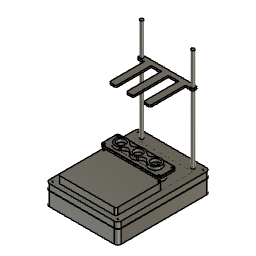
group 5 (Autodesk Fusion 360 design; units mm, degrees)
Autodesk Fusion 360 part; units mm, degrees
note: some values were not read from the file. Chosen so that the rebuilt part matches the saved one: which face or edge a step refers to.
(part 1 of 2)
sketch "Sketch1" plane through (0, 0, 0) normal (0, 0, 1) x (1, 0, 0)
  line L0 (127.613, 86.765) -> (0.7281, 86.765)
  line L1 (127.613, 0.765) -> (127.613, 86.765)
  line L2 (0.7281, 0.765) -> (127.613, 0.765)
  line L3 (0.7281, 86.765) -> (0.7281, 0.765)
  dimension "d1" = 86
  dimension "d2" = 126.8849
  constraint horizontal L0
  constraint vertical L3
  constraint horizontal L2
  constraint vertical L1
  measures "d1" distance of L2.start L0.end
  measures "d2" distance of L0.start L0.end
extrude "Extrude1" add sketch "Sketch1" along normal blind 30 makes body 1
sketch "Sketch2" plane through (0, 0, 30) normal (0, 0, 1) x (-1, 0, 0)
  line L0 (-0.7281, -86.765) -> (-0.7281, -0.765)
  line L1 (-0.7281, -0.765) -> (-127.613, -0.765)
  line L2 (-127.613, -0.765) -> (-127.613, -86.765)
  line L3 (-127.613, -86.765) -> (-0.7281, -86.765)
  circle A0 centre (-30, -70) radius 10
  circle A1 centre (-60, -70) radius 10
  circle A2 centre (-90, -70) radius 10
  circle A3 centre (-30, -30) radius 10
  circle A4 centre (-60, -30) radius 10
  circle A5 centre (-90, -30) radius 10
  point P0 (-30, -70)
  dimension "d5" = 20
  dimension "d6" = 20
  dimension "d7" = 20
  dimension "d8" = 20
  measures "d5" diameter of A2
  measures "d6" diameter of A3
  measures "d7" diameter of A4
  measures "d8" diameter of A5
extrude "Extrude2" cut sketch "Sketch2" against normal blind 10 contours A0 | A1 | A2 | A3 | A4 | A5 bodies 1
sketch "Sketch3" plane through (0, 0, 0) normal (0, 0, 1) x (1, 0, 0)
  circle A0 centre (23.2455, 19.8373) radius 15
  dimension "d11" = 30
  measures "d11" diameter of A0
extrude "Extrude3" add sketch "Sketch3" against normal blind 10 bodies 1
move_face "MoveFace1" to x (1, 0, 0) y (0, 1, 0) z (0, 0, 1) at (0, 0, -20) 1 faces at (38.2269, 19.0896, -6.6667) on bodies 1
move_face "MoveFace2" to x (1, 0, 0) y (0, 1, 0) z (0, 0, 1) at (0, 0, -10) 1 faces at (38.2269, 19.0896, -6.6667) on bodies 1
move_face "MoveFace3" by (0, 0, -15) 1 faces at (27.3111, 19.0921, -10) on bodies 1
move_face "MoveFace4" to x (1, 0, 0) y (0, 1, 0) z (0, 0, 1) at (0, 0, -15) 1 faces at (38.2269, 19.0896, -16.6667) on bodies 1
move_face "MoveFace5" to x (1, 0, 0) y (0, 1, 0) z (0, 0, 1) at (0, 0, -10) 1 faces at (38.2269, 19.0896, -16.6667) on bodies 1
move_face "MoveFace6" to x (1, 0, 0) y (0, 1, 0) z (0, 0, 1) at (0, 0, 15) 1 faces at (38.2269, 19.0896, -16.6667) on bodies 1
split "Split1" by plane through (0, 0, 0) normal (0, 0, -1) bodies 1 makes body 2 at (38.171, 18.3438, -8.3333)
move_face "MoveFace7" to x (1, 0, 0) y (0, 1, 0) z (0, 0, 1) at (0, 0, -20) 1 faces at (38.171, 18.3438, -8.3333) on bodies 2
move_face "MoveFace8" to x (1, 0, 0) y (0, 1, 0) z (0, 0, 1) at (120, 0, -10) 1 faces at (38.171, 18.3438, -8.3333) on bodies 2
extrude "Extrude4" cut 1 faces at (147.3111, 20.5825, 0) along direction (0, 0, -1) blind 10 on bodies 2 bodies 2
move_face "MoveFace9" to x (1, 0, 0) y (0, 1, 0) z (0, 0, 1) at (0, 0, -10) 1 faces at (158.171, 18.3438, -20) on bodies 2
move_body "Move1" bodies 2 to x (1, 0, 0) y (0, 1, 0) z (0, 0, 1) at (0, 0, -20)
sketch "Sketch4" plane through (0, 0, -30) normal (0, 0, 1) x (-1, 0, 0)
  circle A0 centre (-143.2455, -19.8373) radius 15
  circle A1 centre (-143.2455, -19.8373) radius 1
  dimension "d16" = 2
  constraint concentric A0 A1
  measures "d16" diameter of A1
extrude "Extrude5" add sketch "Sketch4" along normal blind 7 contours A1 bodies 2
sketch "Sketch5" plane through (0, 0, -23) normal (0, 0, 1) x (-1, 0, 0)
  circle A0 centre (-143.2455, -19.8373) radius 1
sketch "Sketch6" plane through (0, 0, -23) normal (0, 0, 1) x (1, 0, 0)
sketch "Sketch7" plane through (0, 0, -23) normal (0, 0, 1) x (-1, 0, 0)
  line L0 (-158.0751, -15.2692) -> (-128.1492, -15.2692)
  line L1 (-128.1492, -15.2692) -> (-128.1492, -22.9458)
  line L2 (-128.1492, -22.9458) -> (-158.0751, -22.9458)
  line L3 (-158.0751, -22.9458) -> (-158.0751, -15.2692)
  constraint horizontal L0
  constraint vertical L1
  constraint horizontal L2
  constraint vertical L3
extrude "Extrude6" add sketch "Sketch7" along normal blind 3 bodies 2
sketch "Sketch8" plane through (0, 0, -20) normal (0, 0, 1) x (-1, 0, 0)
  line L0 (-158.0751, -22.9458) -> (-128.1492, -22.9458)
  line L1 (-128.1492, -22.9458) -> (-128.1492, -15.2692)
  line L2 (-128.1492, -15.2692) -> (-158.0751, -15.2692)
  line L3 (-158.0751, -15.2692) -> (-158.0751, -22.9458)
  circle A0 centre (-132.1474, -19.1075) radius 2.5
  circle A1 centre (-154.0063, -18.9019) radius 2.5
  dimension "d21" = 5
  dimension "d22" = 5
  measures "d21" diameter of A0
  measures "d22" diameter of A1
extrude "Extrude7" cut sketch "Sketch8" against normal blind 3 contours A0 | A1 bodies 2
extrude "Extrude8" cut sketch "Sketch5" along normal blind 10 bodies 2
extrude "Extrude9" add 6 faces at (86.9158, 73.324, 20) (57.2459, 67.1287, 20) (27.0978, 72.8603, 20) (35.1448, 31.1294, 20) (63.9941, 31.372, 20) (87.9217, 27.3939, 20) along direction (0, 0, 1) blind 2 on bodies 1 bodies 1
delete_body "RemoveBody1" bodies 1
sketch "Sketch9" plane through (0, 0, 0) normal (0, 0, 1) x (1, 0, 0)
  line L0 (0, 0) -> (-150, 0)
  line L1 (-150, 0) -> (-150, 50)
  line L2 (-150, 50) -> (0, 50)
  line L3 (0, 50) -> (0, 0)
  constraint horizontal L0
  constraint vertical L1
  constraint horizontal L2
  constraint vertical L3
  constraint coincident L0.start L3.end
sketch "Sketch10" plane through (0, 0, 2) normal (0, 0, 1) x (-1, 0, 0)
sketch "Sketch11" plane through (0, 0, 2) normal (0, 0, 1) x (-1, 0, 0)
  arc A0 (148.0002, -49) -> (149, -48.0002) centre (148.0002, -48.0002) ccw
  line L0 (149, -48.0002) -> (149, -1.9998)
  arc A1 (149, -1.9998) -> (148.0002, -1) centre (148.0002, -1.9998) ccw
  line L1 (148.0002, -1) -> (1.9998, -1)
  arc A2 (1.9998, -1) -> (1, -1.9998) centre (1.9998, -1.9998) ccw
  line L2 (1, -1.9998) -> (1, -48.0002)
  arc A3 (1, -48.0002) -> (1.9998, -49) centre (1.9998, -48.0002) ccw
  line L3 (1.9998, -49) -> (148.0002, -49)
sketch "Sketch12" plane through (0, 0, 0) normal (0, 0, 1) x (1, 0, 0)
  line L0 (-165, 50) -> (-5, 50)
  line L1 (0, 45) -> (0, 5)
  line L2 (-5, 0) -> (-165, 0)
  line L3 (-170, 5) -> (-170, 45)
  arc A0 (-165, 50) -> (-170, 45) centre (-165, 45) ccw
  arc A1 (-170, 5) -> (-165, 0) centre (-165, 5) ccw
  arc A2 (-5, 0) -> (0, 5) centre (-5, 5) ccw
  arc A3 (0, 45) -> (-5, 50) centre (-5, 45) ccw
  arc A4 (0, 45) -> (-5, 50) centre (-5, 45) ccw
  dimension "d33" = 5
  dimension "d34" = 5
  dimension "d35" = 5
  dimension "d36" = 5
  dimension "d37" = 5
  constraint horizontal L0
  constraint vertical L1
  constraint horizontal L2
  constraint vertical L3
  constraint tangent L3 A0
  constraint tangent L0 A0
  constraint tangent L3 A1
  constraint tangent L2 A1
  constraint tangent L2 A2
  constraint tangent L1 A2
  constraint tangent L0 A3
  constraint tangent L1 A3
  constraint coincident L0 A3.end
  constraint coincident L1 A3.start
  constraint tangent L0 A4
  constraint tangent L1 A4
  measures "d33" radius of A0
  measures "d34" radius of A1
  measures "d35" radius of A2
  measures "d36" radius of A3
  measures "d37" radius of A4
extrude "Extrude11" add sketch "Sketch12" along normal blind 2 separate body makes body 3
sketch "Sketch13" plane through (0, 0, 2) normal (0, 0, 1) x (-1, 0, 0)
  arc A0 (5, 0) -> (0, -5) centre (5, -5) ccw
  line L0 (0, -5) -> (0, -45)
  arc A1 (0, -45) -> (5, -50) centre (5, -45) ccw
  line L1 (5, -50) -> (165, -50)
  arc A2 (165, -50) -> (170, -45) centre (165, -45) ccw
  line L2 (170, -45) -> (170, -5)
  arc A3 (170, -5) -> (165, 0) centre (165, -5) ccw
  line L3 (165, 0) -> (5, 0)
  circle A4 centre (5, -5) radius 2.5
  circle A5 centre (5, -45) radius 2.5
  circle A6 centre (165, -45) radius 2.5
  circle A7 centre (165, -5) radius 2.5
  dimension "d40" = 5
  dimension "d41" = 5
  dimension "d42" = 5
  dimension "d43" = 5
  constraint concentric A0 A4
  constraint concentric A1 A5
  constraint concentric A2 A6
  constraint concentric A3 A7
  measures "d40" diameter of A4
  measures "d41" diameter of A5
  measures "d42" diameter of A6
  measures "d43" diameter of A7
extrude "Extrude12" cut sketch "Sketch13" against normal blind 22 contours A4 | A5 | A6 | A7 bodies 3
sketch "Sketch14" plane through (0, 0, 2) normal (0, 0, 1) x (-1, 0, 0)
  circle A0 centre (5, -45) radius 2.5
  circle A1 centre (165, -45) radius 2.5
  circle A2 centre (5, -5) radius 2.5
  circle A3 centre (165, -5) radius 2.5
  arc A4 (5, 0) -> (0, -5) centre (5, -5) ccw
  line L0 (0, -5) -> (0, -45)
  arc A5 (0, -45) -> (5, -50) centre (5, -45) ccw
  line L1 (5, -50) -> (165, -50)
  arc A6 (165, -50) -> (170, -45) centre (165, -45) ccw
  line L2 (170, -45) -> (170, -5)
  arc A7 (170, -5) -> (165, 0) centre (165, -5) ccw
  line L3 (165, 0) -> (5, 0)
  circle A8 centre (35, -25) radius 17.5
  circle A9 centre (85, -25) radius 17.5
  circle A10 centre (135, -25) radius 17.5
  spline S0 degree 5 poles (34.8499, -42.4994) (35.2778, -42.6398) (36.1416, -42.8539) (37.4614, -42.9749) (39.2693, -42.7341) (41.6104, -41.7743) (44.0327, -40.2087) (46.5344, -38.1535) (49.1112, -35.8252) (51.7554, -33.5206) (54.457, -31.5586) (57.203, -30.2337) (59.978, -29.7646) (62.7639, -30.243) (65.5399, -31.5793) (68.284, -33.5556) (70.9744, -35.8771) (73.5912, -38.2226) (76.118, -40.2917) (78.5436, -41.8607) (80.8626, -42.8095) (82.6314, -43.0285) (83.9095, -42.8836) (84.7401, -42.6503) (85.1501, -42.4994) knots 0 0 0 0 0 0 0.05 0.1 0.15 0.2 0.25 0.3 0.35 0.4 0.45 0.5 0.55 0.6 0.65 0.7 0.75 0.8 0.85 0.9 0.95 1 1 1 1 1 1
  spline S1 degree 5 poles (35.0693, -7.5001) (35.4803, -7.36) (36.3119, -7.1467) (37.5885, -7.0274) (39.3489, -7.2715) (41.6475, -8.2369) (44.0435, -9.8086) (46.5336, -11.8686) (49.1104, -14.1971) (51.7624, -16.4976) (54.4748, -18.4525) (57.2304, -19.77) (60.0099, -20.2341) (62.7929, -19.7557) (65.5581, -18.425) (68.2846, -16.4587) (70.9525, -14.1493) (73.5443, -11.815) (76.0458, -9.7534) (78.4474, -8.1854) (80.7452, -7.2301) (82.4993, -6.9992) (83.7679, -7.1313) (84.5928, -7.3546) (85, -7.5) knots 0 0 0 0 0 0 0.05 0.1 0.15 0.2 0.25 0.3 0.35 0.4 0.45 0.5 0.55 0.6 0.65 0.7 0.75 0.8 0.85 0.9 0.95 1 1 1 1 1 1
  spline S2 degree 5 poles (35.0693, -7.5001) (35.4803, -7.36) (36.3119, -7.1467) (37.5885, -7.0274) (39.3489, -7.2715) (41.6475, -8.2369) (44.0435, -9.8086) (46.5336, -11.8686) (49.1104, -14.1971) (51.7624, -16.4976) (54.4748, -18.4525) (57.2304, -19.77) (60.0099, -20.2341) (62.7929, -19.7557) (65.5581, -18.425) (68.2846, -16.4587) (70.9525, -14.1493) (73.5443, -11.815) (76.0458, -9.7534) (78.4474, -8.1854) (80.7452, -7.2301) (82.4993, -6.9992) (83.7679, -7.1313) (84.5928, -7.3546) (85, -7.5) knots 0 0 0 0 0 0 0.05 0.1 0.15 0.2 0.25 0.3 0.35 0.4 0.45 0.5 0.55 0.6 0.65 0.7 0.75 0.8 0.85 0.9 0.95 1 1 1 1 1 1
  spline S3 degree 5 poles (84.8499, -42.4994) (85.2778, -42.6398) (86.1416, -42.8539) (87.4614, -42.9749) (89.2693, -42.7341) (91.6104, -41.7743) (94.0327, -40.2087) (96.5344, -38.1535) (99.1112, -35.8252) (101.7554, -33.5206) (104.457, -31.5586) (107.203, -30.2337) (109.978, -29.7646) (112.7639, -30.243) (115.5399, -31.5793) (118.284, -33.5556) (120.9744, -35.8771) (123.5912, -38.2226) (126.118, -40.2917) (128.5436, -41.8607) (130.8626, -42.8095) (132.6314, -43.0285) (133.9095, -42.8836) (134.7401, -42.6503) (135.1501, -42.4994) knots 0 0 0 0 0 0 0.05 0.1 0.15 0.2 0.25 0.3 0.35 0.4 0.45 0.5 0.55 0.6 0.65 0.7 0.75 0.8 0.85 0.9 0.95 1 1 1 1 1 1
  spline S4 degree 5 poles (85.0693, -7.5001) (85.4803, -7.36) (86.3119, -7.1467) (87.5885, -7.0274) (89.3489, -7.2715) (91.6475, -8.2369) (94.0435, -9.8086) (96.5336, -11.8686) (99.1104, -14.1971) (101.7624, -16.4976) (104.4748, -18.4525) (107.2304, -19.77) (110.0099, -20.2341) (112.7929, -19.7557) (115.5581, -18.425) (118.2846, -16.4587) (120.9525, -14.1493) (123.5443, -11.815) (126.0458, -9.7534) (128.4474, -8.1854) (130.7452, -7.2301) (132.4993, -6.9992) (133.7679, -7.1313) (134.5928, -7.3546) (135, -7.5) knots 0 0 0 0 0 0 0.05 0.1 0.15 0.2 0.25 0.3 0.35 0.4 0.45 0.5 0.55 0.6 0.65 0.7 0.75 0.8 0.85 0.9 0.95 1 1 1 1 1 1
  point P0 (45.0607, -39.3189)
  point P1 (60, -30)
  point P2 (75.2634, -39.5413)
  point P3 (75.1901, -10.508)
  point P4 (60, -20)
  point P5 (44.9315, -10.5911)
  point P6 (75.1901, -10.508)
  point P7 (60, -20)
  point P8 (44.9315, -10.5911)
  point P9 (125.2634, -39.5413)
  point P10 (95.0607, -39.3189)
  point P11 (110, -30)
  point P12 (94.9315, -10.5911)
  point P13 (125.1901, -10.508)
  point P14 (110, -20)
  dimension "d46" = 35
  dimension "d47" = 35
  dimension "d48" = 35
  constraint coincident A8 S0.start
  constraint coincident A8 P0
  constraint coincident A9 P2
  constraint coincident A9 S0.end
  constraint coincident A8 P8
  constraint coincident A9 P6
  measures "d46" diameter of A8
  measures "d47" diameter of A9
  measures "d48" diameter of A10
extrude "Extrude13" add sketch "Sketch14" along normal blind 9 contours A8 S0 S1 S2 | A8 A9 S0 S1 S2 | A9 S0 S1 S2 S3 S4 | A9 A10 S3 S4 | A10 S3 S4 bodies 3
sketch "Sketch15" plane through (0, 0, 11) normal (0, 0, 1) x (-1, 0, 0)
  arc A0 (94.9315, -10.5911) -> (75.1901, -10.508) centre (85, -25) ccw
  spline S0 degree 5 poles (75.1901, -10.508) (74.8606, -10.7669) (74.3102, -11.2115) (73.754, -11.6786) (73.1923, -12.1628) (72.6254, -12.658) (72.3993, -12.8562) knots -0.783167 -0.783167 -0.783167 -0.783167 -0.783167 -0.783167 -0.75 -0.728117 -0.728117 -0.728117 -0.728117 -0.728117 -0.728117
  spline S1 degree 5 poles (72.3993, -12.8562) (72.1087, -13.1109) (71.2977, -13.8245) (69.9514, -15.0122) (68.046, -16.6308) (65.5581, -18.425) (62.7929, -19.7557) (60.0099, -20.2341) (57.2304, -19.77) (54.4748, -18.4525) (51.9684, -16.646) (50.0441, -15.0041) (48.6764, -13.7923) (47.8412, -13.0553) (47.523, -12.7761) knots -0.728117 -0.728117 -0.728117 -0.728117 -0.728117 -0.728117 -0.7 -0.65 -0.6 -0.55 -0.5 -0.45 -0.4 -0.35 -0.3 -0.268985 -0.268985 -0.268985 -0.268985 -0.268985 -0.268985
  spline S2 degree 5 poles (47.523, -12.7761) (47.3283, -12.6052) (46.8025, -12.1454) (46.2812, -11.6956) (45.7645, -11.2606) (45.2525, -10.8448) (44.9315, -10.5911) knots -0.268985 -0.268985 -0.268985 -0.268985 -0.268985 -0.268985 -0.25 -0.217579 -0.217579 -0.217579 -0.217579 -0.217579 -0.217579
  arc A1 (44.9315, -10.5911) -> (45.0607, -39.3189) centre (35, -25) ccw
  spline S3 degree 5 poles (45.0607, -39.3189) (45.3565, -39.0848) (45.8139, -38.7136) (46.2744, -38.3276) (46.7381, -37.9297) (47.2049, -37.5233) (47.3687, -37.38) knots 0.220346 0.220346 0.220346 0.220346 0.220346 0.220346 0.25 0.265988 0.265988 0.265988 0.265988 0.265988 0.265988
  spline S4 degree 5 poles (47.3687, -37.38) (47.7173, -37.0753) (48.5825, -36.3127) (49.9785, -35.0712) (51.9282, -33.3951) (54.457, -31.5586) (57.203, -30.2337) (59.978, -29.7646) (62.7639, -30.243) (65.5399, -31.5793) (68.0374, -33.378) (69.9522, -34.999) (71.3047, -36.1869) (72.1174, -36.8988) (72.4048, -37.1495) knots 0.265988 0.265988 0.265988 0.265988 0.265988 0.265988 0.3 0.35 0.4 0.45 0.5 0.55 0.6 0.65 0.7 0.727531 0.727531 0.727531 0.727531 0.727531 0.727531
  spline S5 degree 5 poles (72.4048, -37.1495) (72.6393, -37.3541) (73.2199, -37.859) (73.7952, -38.3525) (74.3649, -38.8281) (74.9287, -39.2804) (75.2634, -39.5413) knots 0.727531 0.727531 0.727531 0.727531 0.727531 0.727531 0.75 0.783359 0.783359 0.783359 0.783359 0.783359 0.783359
  arc A2 (75.2634, -39.5413) -> (95.0607, -39.3189) centre (85, -25) ccw
  spline S6 degree 5 poles (95.0607, -39.3189) (95.3565, -39.0848) (95.8139, -38.7136) (96.2744, -38.3276) (96.7381, -37.9297) (97.2049, -37.5233) (97.3687, -37.38) knots 0.220346 0.220346 0.220346 0.220346 0.220346 0.220346 0.25 0.265988 0.265988 0.265988 0.265988 0.265988 0.265988
  spline S7 degree 5 poles (97.3687, -37.38) (97.7173, -37.0753) (98.5825, -36.3127) (99.9785, -35.0712) (101.9282, -33.3951) (104.457, -31.5586) (107.203, -30.2337) (109.978, -29.7646) (112.7639, -30.243) (115.5399, -31.5793) (118.0374, -33.378) (119.9522, -34.999) (121.3047, -36.1869) (122.1174, -36.8988) (122.4048, -37.1495) knots 0.265988 0.265988 0.265988 0.265988 0.265988 0.265988 0.3 0.35 0.4 0.45 0.5 0.55 0.6 0.65 0.7 0.727531 0.727531 0.727531 0.727531 0.727531 0.727531
  spline S8 degree 5 poles (122.4048, -37.1495) (122.6393, -37.3541) (123.2199, -37.859) (123.7952, -38.3525) (124.3649, -38.8281) (124.9287, -39.2804) (125.2634, -39.5413) knots 0.727531 0.727531 0.727531 0.727531 0.727531 0.727531 0.75 0.783359 0.783359 0.783359 0.783359 0.783359 0.783359
  arc A3 (125.2634, -39.5413) -> (125.1901, -10.508) centre (135, -25) ccw
  spline S9 degree 5 poles (125.1901, -10.508) (124.8606, -10.7669) (124.3102, -11.2115) (123.754, -11.6786) (123.1923, -12.1628) (122.6254, -12.658) (122.3993, -12.8562) knots -0.783167 -0.783167 -0.783167 -0.783167 -0.783167 -0.783167 -0.75 -0.728117 -0.728117 -0.728117 -0.728117 -0.728117 -0.728117
  spline S10 degree 5 poles (122.3993, -12.8562) (122.1087, -13.1109) (121.2977, -13.8245) (119.9514, -15.0122) (118.046, -16.6308) (115.5581, -18.425) (112.7929, -19.7557) (110.0099, -20.2341) (107.2304, -19.77) (104.4748, -18.4525) (101.9684, -16.646) (100.0441, -15.0041) (98.6764, -13.7923) (97.8412, -13.0553) (97.523, -12.7761) knots -0.728117 -0.728117 -0.728117 -0.728117 -0.728117 -0.728117 -0.7 -0.65 -0.6 -0.55 -0.5 -0.45 -0.4 -0.35 -0.3 -0.268985 -0.268985 -0.268985 -0.268985 -0.268985 -0.268985
  spline S11 degree 5 poles (97.523, -12.7761) (97.3283, -12.6052) (96.8025, -12.1454) (96.2812, -11.6956) (95.7645, -11.2606) (95.2525, -10.8448) (94.9315, -10.5911) knots -0.268985 -0.268985 -0.268985 -0.268985 -0.268985 -0.268985 -0.25 -0.217579 -0.217579 -0.217579 -0.217579 -0.217579 -0.217579
  circle A4 centre (35, -25) radius 12.5
  circle A5 centre (85, -25) radius 12.5
  circle A6 centre (135, -25) radius 12.5
  dimension "d51" = 25
  dimension "d52" = 25
  dimension "d53" = 25
  constraint concentric A1 A4
  constraint concentric A0 A5
  constraint concentric A3 A6
  measures "d51" diameter of A4
  measures "d52" diameter of A5
  measures "d53" diameter of A6
extrude "Extrude14" cut sketch "Sketch15" against normal blind 9 contours A4 | A5 | A6 bodies 3
sketch "Sketch16" plane through (0, 0, 0) normal (0, 0, 1) x (1, 0, 0)
sketch "Sketch17" plane through (0, 0, 11) normal (0, 0, 1) x (-1, 0, 0)
  circle A0 centre (35, -25) radius 12.5
  circle A1 centre (85, -25) radius 12.5
  circle A2 centre (135, -25) radius 12.5
  arc A3 (94.9315, -10.5911) -> (75.1901, -10.508) centre (85, -25) ccw
  spline S0 degree 5 poles (75.1901, -10.508) (74.8606, -10.7669) (74.3102, -11.2115) (73.754, -11.6786) (73.1923, -12.1628) (72.6254, -12.658) (72.3993, -12.8562) knots -0.783167 -0.783167 -0.783167 -0.783167 -0.783167 -0.783167 -0.75 -0.728117 -0.728117 -0.728117 -0.728117 -0.728117 -0.728117
  spline S1 degree 5 poles (72.3993, -12.8562) (72.1087, -13.1109) (71.2977, -13.8245) (69.9514, -15.0122) (68.046, -16.6308) (65.5581, -18.425) (62.7929, -19.7557) (60.0099, -20.2341) (57.2304, -19.77) (54.4748, -18.4525) (51.9684, -16.646) (50.0441, -15.0041) (48.6764, -13.7923) (47.8412, -13.0553) (47.523, -12.7761) knots -0.728117 -0.728117 -0.728117 -0.728117 -0.728117 -0.728117 -0.7 -0.65 -0.6 -0.55 -0.5 -0.45 -0.4 -0.35 -0.3 -0.268985 -0.268985 -0.268985 -0.268985 -0.268985 -0.268985
  spline S2 degree 5 poles (47.523, -12.7761) (47.3283, -12.6052) (46.8025, -12.1454) (46.2812, -11.6956) (45.7645, -11.2606) (45.2525, -10.8448) (44.9315, -10.5911) knots -0.268985 -0.268985 -0.268985 -0.268985 -0.268985 -0.268985 -0.25 -0.217579 -0.217579 -0.217579 -0.217579 -0.217579 -0.217579
  arc A4 (44.9315, -10.5911) -> (45.0607, -39.3189) centre (35, -25) ccw
  spline S3 degree 5 poles (45.0607, -39.3189) (45.3565, -39.0848) (45.8139, -38.7136) (46.2744, -38.3276) (46.7381, -37.9297) (47.2049, -37.5233) (47.3687, -37.38) knots 0.220346 0.220346 0.220346 0.220346 0.220346 0.220346 0.25 0.265988 0.265988 0.265988 0.265988 0.265988 0.265988
  spline S4 degree 5 poles (47.3687, -37.38) (47.7173, -37.0753) (48.5825, -36.3127) (49.9785, -35.0712) (51.9282, -33.3951) (54.457, -31.5586) (57.203, -30.2337) (59.978, -29.7646) (62.7639, -30.243) (65.5399, -31.5793) (68.0374, -33.378) (69.9522, -34.999) (71.3047, -36.1869) (72.1174, -36.8988) (72.4048, -37.1495) knots 0.265988 0.265988 0.265988 0.265988 0.265988 0.265988 0.3 0.35 0.4 0.45 0.5 0.55 0.6 0.65 0.7 0.727531 0.727531 0.727531 0.727531 0.727531 0.727531
  spline S5 degree 5 poles (72.4048, -37.1495) (72.6393, -37.3541) (73.2199, -37.859) (73.7952, -38.3525) (74.3649, -38.8281) (74.9287, -39.2804) (75.2634, -39.5413) knots 0.727531 0.727531 0.727531 0.727531 0.727531 0.727531 0.75 0.783359 0.783359 0.783359 0.783359 0.783359 0.783359
  arc A5 (75.2634, -39.5413) -> (95.0607, -39.3189) centre (85, -25) ccw
  spline S6 degree 5 poles (95.0607, -39.3189) (95.3565, -39.0848) (95.8139, -38.7136) (96.2744, -38.3276) (96.7381, -37.9297) (97.2049, -37.5233) (97.3687, -37.38) knots 0.220346 0.220346 0.220346 0.220346 0.220346 0.220346 0.25 0.265988 0.265988 0.265988 0.265988 0.265988 0.265988
  spline S7 degree 5 poles (97.3687, -37.38) (97.7173, -37.0753) (98.5825, -36.3127) (99.9785, -35.0712) (101.9282, -33.3951) (104.457, -31.5586) (107.203, -30.2337) (109.978, -29.7646) (112.7639, -30.243) (115.5399, -31.5793) (118.0374, -33.378) (119.9522, -34.999) (121.3047, -36.1869) (122.1174, -36.8988) (122.4048, -37.1495) knots 0.265988 0.265988 0.265988 0.265988 0.265988 0.265988 0.3 0.35 0.4 0.45 0.5 0.55 0.6 0.65 0.7 0.727531 0.727531 0.727531 0.727531 0.727531 0.727531
  spline S8 degree 5 poles (122.4048, -37.1495) (122.6393, -37.3541) (123.2199, -37.859) (123.7952, -38.3525) (124.3649, -38.8281) (124.9287, -39.2804) (125.2634, -39.5413) knots 0.727531 0.727531 0.727531 0.727531 0.727531 0.727531 0.75 0.783359 0.783359 0.783359 0.783359 0.783359 0.783359
  arc A6 (125.2634, -39.5413) -> (125.1901, -10.508) centre (135, -25) ccw
  spline S9 degree 5 poles (125.1901, -10.508) (124.8606, -10.7669) (124.3102, -11.2115) (123.754, -11.6786) (123.1923, -12.1628) (122.6254, -12.658) (122.3993, -12.8562) knots -0.783167 -0.783167 -0.783167 -0.783167 -0.783167 -0.783167 -0.75 -0.728117 -0.728117 -0.728117 -0.728117 -0.728117 -0.728117
  spline S10 degree 5 poles (122.3993, -12.8562) (122.1087, -13.1109) (121.2977, -13.8245) (119.9514, -15.0122) (118.046, -16.6308) (115.5581, -18.425) (112.7929, -19.7557) (110.0099, -20.2341) (107.2304, -19.77) (104.4748, -18.4525) (101.9684, -16.646) (100.0441, -15.0041) (98.6764, -13.7923) (97.8412, -13.0553) (97.523, -12.7761) knots -0.728117 -0.728117 -0.728117 -0.728117 -0.728117 -0.728117 -0.7 -0.65 -0.6 -0.55 -0.5 -0.45 -0.4 -0.35 -0.3 -0.268985 -0.268985 -0.268985 -0.268985 -0.268985 -0.268985
  spline S11 degree 5 poles (97.523, -12.7761) (97.3283, -12.6052) (96.8025, -12.1454) (96.2812, -11.6956) (95.7645, -11.2606) (95.2525, -10.8448) (94.9315, -10.5911) knots -0.268985 -0.268985 -0.268985 -0.268985 -0.268985 -0.268985 -0.25 -0.217579 -0.217579 -0.217579 -0.217579 -0.217579 -0.217579
sketch "Sketch18" plane through (0, 0, 0) normal (0, 0, -1) x (1, 0, 0)
  arc A0 (0, -5) -> (-5, 0) centre (-5, -5) ccw
  line L0 (-5, 0) -> (-165, 0)
  arc A1 (-165, 0) -> (-170, -5) centre (-165, -5) ccw
  line L1 (-170, -5) -> (-170, -45)
  arc A2 (-170, -45) -> (-165, -50) centre (-165, -45) ccw
  line L2 (-165, -50) -> (-5, -50)
  arc A3 (-5, -50) -> (0, -45) centre (-5, -45) ccw
  line L3 (0, -45) -> (0, -5)
  circle A4 centre (-5, -45) radius 2.5
  circle A5 centre (-165, -45) radius 2.5
  circle A6 centre (-5, -5) radius 2.5
  circle A7 centre (-165, -5) radius 2.5
sketch "Sketch19" plane through (0, 0, 0) normal (0, 0, -1) x (1, 0, 0)
sketch "Sketch20" plane through (0, 0, 0) normal (0, 0, 1) x (1, 0, 0)
sketch "Sketch21" plane through (0, 0, 0) normal (0, 0, -1) x (1, 0, 0)
  line L0 (-165, -10) -> (-5, -10)
  line L1 (0, -5) -> (0, 120)
  line L2 (-5, 125) -> (-165, 125)
  line L3 (-170, 120) -> (-170, -5)
  arc A0 (-165, 125) -> (-170, 120) centre (-165, 120) ccw
  arc A1 (0, 120) -> (-5, 125) centre (-5, 120) ccw
  arc A2 (-170, -5) -> (-165, -10) centre (-165, -5) ccw
  arc A3 (-5, -10) -> (0, -5) centre (-5, -5) ccw
  dimension "d56" = 5
  dimension "d57" = 5
  dimension "d58" = 5
  dimension "d59" = 5
  constraint horizontal L0
  constraint vertical L1
  constraint horizontal L2
  constraint vertical L3
  constraint tangent L2 A0
  constraint tangent L3 A0
  constraint tangent L2 A1
  constraint tangent L1 A1
  constraint tangent L3 A2
  constraint tangent L0 A2
  constraint tangent L1 A3
  constraint tangent L0 A3
  measures "d56" radius of A0
  measures "d57" radius of A1
  measures "d58" radius of A2
  measures "d59" radius of A3
extrude "Extrude15" add sketch "Sketch21" along normal blind 20 bodies 3
extrude "Extrude16" cut sketch "Sketch14" against normal blind 22 contours A2 bodies 3
extrude "Extrude17" cut sketch "Sketch14" against normal blind 22 contours A3 bodies 3
sketch "Sketch22" plane through (0, 0, -20) normal (0, 0, -1) x (1, 0, 0)
  circle A0 centre (-165, -5) radius 2.5
  circle A1 centre (-5, -5) radius 2.5
  arc A2 (-5, -10) -> (0, -5) centre (-5, -5) ccw
  line L0 (0, -5) -> (0, 120)
  arc A3 (0, 120) -> (-5, 125) centre (-5, 120) ccw
  line L1 (-5, 125) -> (-165, 125)
  arc A4 (-165, 125) -> (-170, 120) centre (-165, 120) ccw
  line L2 (-170, 120) -> (-170, -5)
  arc A5 (-170, -5) -> (-165, -10) centre (-165, -5) ccw
  line L3 (-165, -10) -> (-5, -10)
  line L4 (-180, 140) -> (10, 140)
  line L5 (20, 130) -> (20, -120)
  line L6 (10, -130) -> (-180, -130)
  line L7 (-190, -120) -> (-190, 130)
  arc A6 (-180, 140) -> (-190, 130) centre (-180, 130) ccw
  arc A7 (20, 130) -> (10, 140) centre (10, 130) ccw
  arc A8 (-190, -120) -> (-180, -130) centre (-180, -120) ccw
  arc A9 (10, -130) -> (20, -120) centre (10, -120) ccw
  circle A10 centre (-180, 130) radius 3.5
  circle A11 centre (10, 130) radius 3.5
  circle A12 centre (-180, -120) radius 3.5
  circle A13 centre (10, -120) radius 3.5
  circle A14 centre (-180, 130) radius 1.75
  circle A15 centre (10, 130) radius 1.75
  circle A16 centre (10, -120) radius 1.75
  circle A17 centre (-180, -120) radius 1.75
  dimension "d66" = 10
  dimension "d67" = 10
  dimension "d68" = 10
  dimension "d69" = 10
  dimension "d70" = 7
  dimension "d71" = 3.5
  dimension "d72" = 3.5
  dimension "d73" = 3.5
  dimension "d74" = 3.5
  constraint horizontal L4
  constraint vertical L5
  constraint horizontal L6
  constraint vertical L7
  constraint tangent L4 A6
  constraint tangent L7 A6
  constraint tangent L4 A7
  constraint tangent L5 A7
  constraint tangent L7 A8
  constraint tangent L6 A8
  constraint tangent L5 A9
  constraint tangent L6 A9
  constraint concentric A6 A10
  constraint concentric A7 A11
  constraint concentric A8 A12
  constraint concentric A9 A13
  constraint equal A10 A11
  constraint equal A11 A13
  constraint equal A12 A13
  constraint concentric A6 A14
  constraint concentric A7 A15
  constraint concentric A9 A16
  constraint concentric A8 A17
  measures "d66" radius of A6
  measures "d67" radius of A7
  measures "d68" radius of A8
  measures "d69" radius of A9
  measures "d70" diameter of A10
  measures "d71" diameter of A14
  measures "d72" diameter of A15
  measures "d73" diameter of A16
  measures "d74" diameter of A17
extrude "Extrude18" add sketch "Sketch22" along normal blind 17.5 separate body contours L4 L5 L6 L7 A6 A7 A8 A9 | A10 | A11 | A12 | A13 makes body 4
sketch "Sketch23" plane through (0, 0, -37.5) normal (0, 0, -1) x (1, 0, 0)
  circle A0 centre (10, -120) radius 1.75
  line L0 (-5, -10) -> (-165, -10)
  arc A1 (-170, -5) -> (-165, -10) centre (-165, -5) ccw
  line L1 (-170, -5) -> (-170, 120)
  arc A2 (-165, 125) -> (-170, 120) centre (-165, 120) ccw
  line L2 (-165, 125) -> (-5, 125)
  arc A3 (0, 120) -> (-5, 125) centre (-5, 120) ccw
  line L3 (0, 120) -> (0, -5)
  arc A4 (-5, -10) -> (0, -5) centre (-5, -5) ccw
  circle A5 centre (-180, -120) radius 1.75
  circle A6 centre (10, 130) radius 1.75
  circle A7 centre (-180, 130) radius 1.75
  arc A8 (-190, -120) -> (-180, -130) centre (-180, -120) ccw
  line L4 (-180, -130) -> (10, -130)
  arc A9 (10, -130) -> (20, -120) centre (10, -120) ccw
  line L5 (20, -120) -> (20, 130)
  arc A10 (20, 130) -> (10, 140) centre (10, 130) ccw
  line L6 (10, 140) -> (-180, 140)
  arc A11 (-180, 140) -> (-190, 130) centre (-180, 130) ccw
  line L7 (-190, 130) -> (-190, -120)
  line L8 (0, -100) -> (-170, -100)
  line L9 (-170, -100) -> (-170, 120)
  line L10 (-170, 120) -> (0, 120)
  line L11 (0, 120) -> (0, -100)
  constraint horizontal L8
  constraint vertical L9
  constraint horizontal L10
  constraint vertical L11
  constraint coincident L1.end A2.end
extrude "Extrude19" cut sketch "Sketch23" against normal blind 15 contours L0 A1 A4 L8 L9 L11 | L0 A1 L1 L3 A4 L9 L10 L11 bodies 4
sketch "Sketch24" plane through (0, 0, -37.5) normal (0, 0, -1) x (1, 0, 0)
  line L0 (-170, -100) -> (-170, 120)
  arc A0 (-165, 125) -> (-170, 120) centre (-165, 120) ccw
  line L1 (-165, 125) -> (-5, 125)
  arc A1 (0, 120) -> (-5, 125) centre (-5, 120) ccw
  line L2 (0, 120) -> (0, -100)
  line L3 (0, -100) -> (-170, -100)
  circle A2 centre (10, -120) radius 1.75
  circle A3 centre (-180, -120) radius 1.75
  circle A4 centre (10, 130) radius 1.75
  circle A5 centre (-180, 130) radius 1.75
  arc A6 (-190, -120) -> (-180, -130) centre (-180, -120) ccw
  line L4 (-180, -130) -> (10, -130)
  arc A7 (10, -130) -> (20, -120) centre (10, -120) ccw
  line L5 (20, -120) -> (20, 130)
  arc A8 (20, 130) -> (10, 140) centre (10, 130) ccw
  line L6 (10, 140) -> (-180, 140)
  arc A9 (-180, 140) -> (-190, 130) centre (-180, 130) ccw
  line L7 (-190, 130) -> (-190, -120)
  line L8 (-180, -130) -> (10, -130)
  line L9 (20, -120) -> (20, 130)
  line L10 (10, 140) -> (-180, 140)
  line L11 (-190, 130) -> (-190, -120)
  arc A10 (20, 130) -> (10, 140) centre (10, 130) ccw
  arc A11 (-180, 140) -> (-190, 130) centre (-180, 130) ccw
  arc A12 (-190, -120) -> (-180, -130) centre (-180, -120) ccw
  arc A13 (10, -130) -> (20, -120) centre (10, -120) ccw
  line L12 (-170, -100) -> (-170, 120)
  arc A14 (-165, 125) -> (-170, 120) centre (-165, 120) ccw
  line L13 (-165, 125) -> (-5, 125)
  arc A15 (0, 120) -> (-5, 125) centre (-5, 120) ccw
  line L14 (0, 120) -> (0, -100)
  line L15 (0, -100) -> (-170, -100)
  circle A16 centre (10, -120) radius 1.75
  circle A17 centre (-180, -120) radius 1.75
  circle A18 centre (10, 130) radius 1.75
  circle A19 centre (-180, 130) radius 1.75
  arc A20 (-190, -120) -> (-180, -130) centre (-180, -120) ccw
  line L16 (-180, -130) -> (10, -130)
  arc A21 (10, -130) -> (20, -120) centre (10, -120) ccw
  line L17 (20, -120) -> (20, 130)
  arc A22 (20, 130) -> (10, 140) centre (10, 130) ccw
  line L18 (10, 140) -> (-180, 140)
  arc A23 (-180, 140) -> (-190, 130) centre (-180, 130) ccw
  line L19 (-190, 130) -> (-190, -120)
  dimension "d79" = 10
  dimension "d80" = 10
  dimension "d81" = 10
  dimension "d82" = 10
  constraint horizontal L8
  constraint vertical L9
  constraint horizontal L10
  constraint vertical L11
  constraint tangent L9 A10
  constraint tangent L10 A10
  constraint tangent L10 A11
  constraint tangent L11 A11
  constraint tangent L11 A12
  constraint tangent L8 A12
  constraint tangent L8 A13
  constraint tangent L9 A13
  measures "d79" radius of A10
  measures "d80" radius of A11
  measures "d81" radius of A12
  measures "d82" radius of A13
extrude "Extrude20" add sketch "Sketch24" along normal blind 38 from surface at 1 separate body makes body 5
sketch "Sketch25" plane through (0, 0, -76.5) normal (0, 0, -1) x (1, 0, 0)
  circle A0 centre (10, -120) radius 1.75
  circle A1 centre (-180, 130) radius 1.75
  circle A2 centre (-180, -120) radius 1.75
  circle A3 centre (10, 130) radius 1.75
  arc A4 (0, 120) -> (-5, 125) centre (-5, 120) ccw
  line L0 (0, 120) -> (0, -100)
  line L1 (0, -100) -> (-170, -100)
  line L2 (-170, -100) -> (-170, 120)
  arc A5 (-165, 125) -> (-170, 120) centre (-165, 120) ccw
  line L3 (-165, 125) -> (-5, 125)
  line L4 (-190, 130) -> (-190, -120)
  arc A6 (-190, -120) -> (-180, -130) centre (-180, -120) ccw
  line L5 (-180, -130) -> (10, -130)
  arc A7 (10, -130) -> (20, -120) centre (10, -120) ccw
  line L6 (20, -120) -> (20, 130)
  arc A8 (20, 130) -> (10, 140) centre (10, 130) ccw
  line L7 (10, 140) -> (-180, 140)
  arc A9 (-180, 140) -> (-190, 130) centre (-180, 130) ccw
extrude "Extrude21" add sketch "Sketch25" along normal blind 2 contours A4 L0 L1 L2 A5 L3 | L4 A6 L5 A7 L6 A8 L7 A9 bodies 5
sketch "Sketch26" plane through (0, 130, 0) normal (0, 1, 0) x (-1, 0, 0)
  line L0 (180, -38.5) -> (-10, -38.5)
  line L1 (-10, -38.5) -> (-10, -78.5)
  line L2 (-10, -78.5) -> (180, -78.5)
  line L3 (180, -78.5) -> (180, -38.5)
  circle A0 centre (50, -60) radius 5.75
  dimension "d88" = 11.5
  measures "d88" diameter of A0
extrude "Extrude22" cut sketch "Sketch26" against normal blind 30 contours A0 bodies 5
sketch "Sketch27" plane through (0, 0, -76.5) normal (0, 0, 1) x (-1, 0, 0)
  line L0 (165, 125) -> (5, 125)
  arc A0 (5, 125) -> (0, 120) centre (5, 120) ccw
  line L1 (0, 120) -> (0, -100)
  line L2 (0, -100) -> (170, -100)
  line L3 (170, -100) -> (170, 120)
  arc A1 (170, 120) -> (165, 125) centre (165, 120) ccw
sketch "Sketch28" plane through (0, 0, -76.5) normal (0, 0, 1) x (1, 0, 0)
  line L0 (-20, -110) -> (-150, -110)
  line L1 (-160, -100) -> (-160, 80)
  line L2 (-150, 90) -> (-20, 90)
  line L3 (-10, 80) -> (-10, -100)
  arc A0 (-20, -110) -> (-10, -100) centre (-20, -100) ccw
  arc A1 (-160, -100) -> (-150, -110) centre (-150, -100) ccw
  arc A2 (-10, 80) -> (-20, 90) centre (-20, 80) ccw
  arc A3 (-150, 90) -> (-160, 80) centre (-150, 80) ccw
  dimension "d91" = 10
  dimension "d92" = 10
  dimension "d93" = 10
  dimension "d94" = 10
  constraint horizontal L0
  constraint vertical L1
  constraint horizontal L2
  constraint vertical L3
  constraint tangent L0 A0
  constraint tangent L3 A0
  constraint tangent L0 A1
  constraint tangent L1 A1
  constraint tangent L3 A2
  constraint tangent L2 A2
  constraint tangent L2 A3
  constraint tangent L1 A3
  measures "d91" radius of A0
  measures "d92" radius of A1
  measures "d93" radius of A2
  measures "d94" radius of A3
extrude "Extrude23" add sketch "Sketch28" along normal blind 2 from surface at 2 separate body makes body 6
move_body "Move2" bodies 2 to x (1, 0, 0) y (0, 1, 0) z (0, 0, 1) at (-166, 40, 25)
extrude "Extrude24" cut 1 faces at (-18.7896, 61.9254, -20) along direction (0, 0, 1) blind 2 on bodies 2 bodies 2
split "Split2" by plane through (0, 0, 0) normal (0, 0, 1) bodies 3 makes body 7 at (-59.1296, 21.421, 0)
move_body "Move3" bodies 7 to x (1, 0, 0) y (0, 1, 0) z (0, 0, 1) at (0, 0, 4)
move_body "Move4" bodies 7 to x (1, 0, 0) y (0, 1, 0) z (0, 0, 1) at (0, 0, 5)
move_body "Move5" bodies 2 to x (1, 0, 0) y (0, 1, 0) z (0, 0, 1) at (0, -25, 0)
move_body "Move6" bodies 7 to x (1, 0, 0) y (0, 1, 0) z (0, 0, 1) at (0, 0, 5)
sketch "Sketch29" plane through (0, 0, 14) normal (0, 0, -1) x (1, 0, 0)
  circle A0 centre (-5, -5) radius 2.5
  circle A1 centre (-165, -5) radius 2.5
  arc A2 (0, -5) -> (-5, 0) centre (-5, -5) ccw
  line L0 (-5, 0) -> (-165, 0)
  arc A3 (-165, 0) -> (-170, -5) centre (-165, -5) ccw
  line L1 (-170, -5) -> (-170, -45)
  arc A4 (-170, -45) -> (-165, -50) centre (-165, -45) ccw
  line L2 (-165, -50) -> (-5, -50)
  arc A5 (-5, -50) -> (0, -45) centre (-5, -45) ccw
  line L3 (0, -45) -> (0, -5)
  circle A6 centre (-165, -45) radius 2.5
  circle A7 centre (-5, -45) radius 2.5
extrude "Extrude25" add sketch "Sketch29" along normal blind 5 separate body makes body 8
sketch "Sketch30" plane through (0, 0, 14) normal (0, 0, 1) x (-1, 0, 0)
  circle A0 centre (5, -45) radius 2.5
  circle A1 centre (5, -5) radius 2.5
  circle A2 centre (165, -5) radius 2.5
  circle A3 centre (165, -45) radius 2.5
  line L0 (0, -5) -> (0, -45)
  arc A4 (0, -45) -> (5, -50) centre (5, -45) ccw
  line L1 (5, -50) -> (165, -50)
  arc A5 (165, -50) -> (170, -45) centre (165, -45) ccw
  line L2 (170, -45) -> (170, -5)
  arc A6 (170, -5) -> (165, 0) centre (165, -5) ccw
  line L3 (165, 0) -> (5, 0)
  arc A7 (5, 0) -> (0, -5) centre (5, -5) ccw
  line L4 (150, -40) -> (20, -40)
  line L5 (20, -40) -> (20, -10)
  line L6 (20, -10) -> (150, -10)
  line L7 (150, -10) -> (150, -40)
  constraint horizontal L4
  constraint vertical L5
  constraint horizontal L6
  constraint vertical L7
extrude "Extrude26" cut sketch "Sketch30" against normal blind 4 contours L4 L5 L6 L7 bodies 8
sketch "Sketch31" plane through (0, 0, 10) normal (0, 0, 1) x (-1, 0, 0)
  line L0 (150, -10) -> (20, -10)
  line L1 (20, -10) -> (20, -40)
  line L2 (20, -40) -> (150, -40)
  line L3 (150, -40) -> (150, -10)
  spline S0 degree 5 poles (145, -35) (144.3, -35.1373) (142.9329, -35.3545) (140.9813, -35.5086) (138.5772, -35.3701) (135.9005, -34.6387) (133.5466, -33.3941) (131.5038, -31.7279) (129.7521, -29.7931) (128.2608, -27.8224) (126.9865, -26.136) (125.8723, -25.0499) (124.8468, -24.7975) (123.8227, -25.4371) (122.6976, -26.7886) (121.3711, -28.5465) (119.76, -30.368) (117.8155, -31.9792) (115.5349, -33.2504) (112.9516, -34.149) (110.1274, -34.7084) (107.1441, -34.9895) (104.0953, -35.0488) (101.0785, -34.8966) (98.1867, -34.4808) (95.5029, -33.7328) (93.0935, -32.5999) (91.0017, -31.0861) (89.2414, -29.2827) (87.7897, -27.4201) (86.5862, -25.8497) (85.5453, -24.9157) (84.565, -24.8645) (83.5372, -25.7115) (82.3577, -27.2274) (80.9369, -29.0741) (79.21, -30.8949) (77.1498, -32.4423) (74.7688, -33.6148) (72.1096, -34.4016) (69.2387, -34.8529) (66.2388, -35.038) (63.2018, -35.0123) (60.2217, -34.7708) (57.3876, -34.2553) (54.7777, -33.3999) (52.4526, -32.163) (50.4491, -30.569) (48.7741, -28.7375) (47.3963, -26.9373) (46.251, -25.5221) (45.2483, -24.8125) (44.2817, -25.0061) (43.2348, -26.0508) (41.9955, -27.6959) (40.4719, -29.6054) (38.6069, -31.4443) (36.3968, -32.9911) (33.8833, -34.1348) (31.1383, -34.8437) (28.2513, -35.1441) (25.3159, -35.0938) (22.4163, -34.7596) (19.6136, -34.1905) (16.9479, -33.4191) (14.4432, -32.465) (12.5776, -31.5636) (11.2579, -30.8114) (10.4134, -30.2761) (10, -30) knots 0 0 0 0 0 0 0.01538462 0.03076923 0.04615385 0.06153846 0.07692308 0.09230769 0.10769231 0.12307692 0.13846154 0.15384615 0.16923077 0.18461538 0.2 0.21538462 0.23076923 0.24615385 0.26153846 0.27692308 0.29230769 0.30769231 0.32307692 0.33846154 0.35384615 0.36923077 0.38461538 0.4 0.41538462 0.43076923 0.44615385 0.46153846 0.47692308 0.49230769 0.50769231 0.52307692 0.53846154 0.55384615 0.56923077 0.58461538 0.6 0.61538462 0.63076923 0.64615385 0.66153846 0.67692308 0.69230769 0.70769231 0.72307692 0.73846154 0.75384615 0.76923077 0.78461538 0.8 0.81538462 0.83076923 0.84615385 0.86153846 0.87692308 0.89230769 0.90769231 0.92307692 0.93846154 0.95384615 0.96923077 0.98461538 1 1 1 1 1 1
  spline S1 degree 5 poles (145, -35) (144.3, -35.1373) (142.9329, -35.3545) (140.9813, -35.5086) (138.5772, -35.3701) (135.9005, -34.6387) (133.5466, -33.3941) (131.5038, -31.7279) (129.7521, -29.7931) (128.2608, -27.8224) (126.9865, -26.136) (125.8723, -25.0499) (124.8468, -24.7975) (123.8227, -25.4371) (122.6976, -26.7886) (121.3711, -28.5465) (119.76, -30.368) (117.8155, -31.9792) (115.5349, -33.2504) (112.9516, -34.149) (110.1274, -34.7084) (107.1441, -34.9895) (104.0953, -35.0488) (101.0785, -34.8966) (98.1867, -34.4808) (95.5029, -33.7328) (93.0935, -32.5999) (91.0017, -31.0861) (89.2414, -29.2827) (87.7897, -27.4201) (86.5862, -25.8497) (85.5453, -24.9157) (84.565, -24.8645) (83.5372, -25.7115) (82.3577, -27.2274) (80.9369, -29.0741) (79.21, -30.8949) (77.1498, -32.4423) (74.7688, -33.6148) (72.1096, -34.4016) (69.2387, -34.8529) (66.2388, -35.038) (63.2018, -35.0123) (60.2217, -34.7708) (57.3876, -34.2553) (54.7777, -33.3999) (52.4526, -32.163) (50.4491, -30.569) (48.7741, -28.7375) (47.3963, -26.9373) (46.251, -25.5221) (45.2483, -24.8125) (44.2817, -25.0061) (43.2348, -26.0508) (41.9955, -27.6959) (40.4719, -29.6054) (38.6069, -31.4443) (36.3968, -32.9911) (33.8833, -34.1348) (31.1383, -34.8437) (28.2513, -35.1441) (25.3159, -35.0938) (22.4163, -34.7596) (19.6136, -34.1905) (16.9479, -33.4191) (14.4432, -32.465) (12.5776, -31.5636) (11.2579, -30.8114) (10.4134, -30.2761) (10, -30) knots 0 0 0 0 0 0 0.01538462 0.03076923 0.04615385 0.06153846 0.07692308 0.09230769 0.10769231 0.12307692 0.13846154 0.15384615 0.16923077 0.18461538 0.2 0.21538462 0.23076923 0.24615385 0.26153846 0.27692308 0.29230769 0.30769231 0.32307692 0.33846154 0.35384615 0.36923077 0.38461538 0.4 0.41538462 0.43076923 0.44615385 0.46153846 0.47692308 0.49230769 0.50769231 0.52307692 0.53846154 0.55384615 0.56923077 0.58461538 0.6 0.61538462 0.63076923 0.64615385 0.66153846 0.67692308 0.69230769 0.70769231 0.72307692 0.73846154 0.75384615 0.76923077 0.78461538 0.8 0.81538462 0.83076923 0.84615385 0.86153846 0.87692308 0.89230769 0.90769231 0.92307692 0.93846154 0.95384615 0.96923077 0.98461538 1 1 1 1 1 1
  spline S2 degree 5 poles (165, -15.3397) (164.3, -15.2025) (162.9329, -14.9852) (160.9813, -14.8312) (158.5772, -14.9696) (155.9005, -15.701) (153.5466, -16.9456) (151.5038, -18.6118) (149.7521, -20.5466) (148.2608, -22.5173) (146.9865, -24.2038) (145.8723, -25.2898) (144.8468, -25.5422) (143.8227, -24.9026) (142.6976, -23.5511) (141.3711, -21.7932) (139.76, -19.9717) (137.8155, -18.3606) (135.5349, -17.0893) (132.9516, -16.1907) (130.1274, -15.6314) (127.1441, -15.3502) (124.0953, -15.2909) (121.0785, -15.4431) (118.1867, -15.8589) (115.5029, -16.6069) (113.0935, -17.7399) (111.0017, -19.2536) (109.2414, -21.057) (107.7897, -22.9196) (106.5862, -24.49) (105.5453, -25.424) (104.565, -25.4752) (103.5372, -24.6282) (102.3577, -23.1123) (100.9369, -21.2656) (99.21, -19.4448) (97.1498, -17.8974) (94.7688, -16.725) (92.1096, -15.9381) (89.2387, -15.4868) (86.2388, -15.3017) (83.2018, -15.3274) (80.2217, -15.5689) (77.3876, -16.0844) (74.7777, -16.9399) (72.4526, -18.1767) (70.4491, -19.7707) (68.7741, -21.6022) (67.3963, -23.4024) (66.251, -24.8176) (65.2483, -25.5273) (64.2817, -25.3336) (63.2348, -24.2889) (61.9955, -22.6438) (60.4719, -20.7343) (58.6069, -18.8954) (56.3968, -17.3486) (53.8833, -16.2049) (51.1383, -15.496) (48.2513, -15.1956) (45.3159, -15.2459) (42.4163, -15.5801) (39.6136, -16.1492) (36.9479, -16.9207) (34.4432, -17.8748) (32.5776, -18.7762) (31.2579, -19.5283) (30.4134, -20.0636) (30, -20.3397) knots 0 0 0 0 0 0 0.01538462 0.03076923 0.04615385 0.06153846 0.07692308 0.09230769 0.10769231 0.12307692 0.13846154 0.15384615 0.16923077 0.18461538 0.2 0.21538462 0.23076923 0.24615385 0.26153846 0.27692308 0.29230769 0.30769231 0.32307692 0.33846154 0.35384615 0.36923077 0.38461538 0.4 0.41538462 0.43076923 0.44615385 0.46153846 0.47692308 0.49230769 0.50769231 0.52307692 0.53846154 0.55384615 0.56923077 0.58461538 0.6 0.61538462 0.63076923 0.64615385 0.66153846 0.67692308 0.69230769 0.70769231 0.72307692 0.73846154 0.75384615 0.76923077 0.78461538 0.8 0.81538462 0.83076923 0.84615385 0.86153846 0.87692308 0.89230769 0.90769231 0.92307692 0.93846154 0.95384615 0.96923077 0.98461538 1 1 1 1 1 1
  spline S3 degree 5 poles (30, -20.3397) (29.8, -20.6932) (29.4, -21.3693) (28.8, -22.2908) (28, -23.3312) (27, -24.2966) (26, -24.897) (25, -25.1025) (24, -24.897) (23, -24.2966) (22, -23.3312) (21.2, -22.2908) (20.6, -21.3693) (20.2, -20.6932) (20, -20.3397) knots 0 0 0 0 0 0 0.1 0.2 0.3 0.4 0.5 0.6 0.7 0.8 0.9 1 1 1 1 1 1
  spline S4 degree 5 poles (145, -35) (145.654, -35.0144) (146.9343, -35.0149) (148.7714, -34.9305) (151.0532, -34.6467) (153.6197, -34.0038) (155.8947, -33.0789) (157.8771, -31.8942) (159.5756, -30.499) (161.0142, -28.9783) (162.2414, -27.4697) (163.3239, -26.1479) (164.3336, -25.194) (165.3373, -24.7716) (166.3843, -24.9926) (167.5006, -25.9043) (168.4586, -27.1957) (169.2148, -28.477) (169.7355, -29.4693) (170, -30) knots 0 0 0 0 0 0 0.066667 0.133333 0.2 0.266667 0.333333 0.4 0.466667 0.533333 0.6 0.666667 0.733333 0.8 0.866667 0.933333 1 1 1 1 1 1
  line L4 (145, -40) -> (145, -10)
  line L5 (25, -40) -> (25, -10)
  point P0 (130, -30)
  point P1 (125, -25)
  point P2 (120, -30)
  point P3 (105, -35)
  point P4 (90, -30)
  point P5 (85, -25)
  point P6 (80, -30)
  point P7 (65, -35)
  point P8 (50, -30)
  point P9 (45, -25)
  point P10 (40, -30)
  point P11 (25, -35)
  point P12 (90, -30)
  point P13 (120, -30)
  point P14 (25, -35)
  point P15 (125, -25)
  point P16 (105, -35)
  point P17 (65, -35)
  point P18 (40, -30)
  point P19 (50, -30)
  point P20 (45, -25)
  point P21 (130, -30)
  point P22 (85, -25)
  point P23 (80, -30)
  point P24 (110, -20.3397)
  point P25 (140, -20.3397)
  point P26 (45, -15.3397)
  point P27 (145, -25.3397)
  point P28 (125, -15.3397)
  point P29 (85, -15.3397)
  point P30 (60, -20.3397)
  point P31 (70, -20.3397)
  point P32 (65, -25.3397)
  point P33 (150, -20.3397)
  point P34 (105, -25.3397)
  point P35 (100, -20.3397)
  point P36 (25, -25)
  point P37 (160, -30)
  point P38 (165, -25)
  constraint coincident L1 S3.end
  constraint coincident S0.start S1.start
  constraint coincident L2 L4.start
  constraint coincident L0 L4.end
  constraint perpendicular L0 L4
  constraint coincident L0 L5.end
  constraint perpendicular L0 L5
extrude "Extrude27" add sketch "Sketch31" along normal blind 2 separate body contours S0 S1 S2 S3 L4 L5 makes body 9
sketch "Sketch32" plane through (0, 0, 14) normal (0, 0, 1) x (-1, 0, 0)
  line L0 (20, -40) -> (20, -10)
  line L1 (20, -10) -> (150, -10)
  line L2 (150, -10) -> (150, -40)
  line L3 (150, -40) -> (20, -40)
  circle A0 centre (5, -45) radius 2.5
  circle A1 centre (5, -5) radius 2.5
  circle A2 centre (165, -5) radius 2.5
  circle A3 centre (165, -45) radius 2.5
  line L4 (0, -5) -> (0, -45)
  arc A4 (0, -45) -> (5, -50) centre (5, -45) ccw
  line L5 (5, -50) -> (165, -50)
  arc A5 (165, -50) -> (170, -45) centre (165, -45) ccw
  line L6 (170, -45) -> (170, -5)
  arc A6 (170, -5) -> (165, 0) centre (165, -5) ccw
  line L7 (165, 0) -> (5, 0)
  arc A7 (5, 0) -> (0, -5) centre (5, -5) ccw
  line L8 (165, -50) -> (5, -50)
  line L9 (0, -45) -> (0, -5)
  line L10 (5, 0) -> (165, 0)
  line L11 (170, -5) -> (170, -45)
  arc A8 (165, -50) -> (170, -45) centre (165, -45) ccw
  arc A9 (170, -5) -> (165, 0) centre (165, -5) ccw
  arc A10 (0, -45) -> (5, -50) centre (5, -45) ccw
  arc A11 (5, 0) -> (0, -5) centre (5, -5) ccw
  dimension "d106" = 5
  dimension "d107" = 5
  dimension "d108" = 5
  dimension "d109" = 5
  constraint horizontal L8
  constraint vertical L9
  constraint horizontal L10
  constraint vertical L11
  constraint tangent L8 A8
  constraint tangent L11 A8
  constraint tangent L11 A9
  constraint tangent L10 A9
  constraint tangent L8 A10
  constraint tangent L9 A10
  constraint tangent L9 A11
  constraint tangent L10 A11
  measures "d106" radius of A8
  measures "d107" radius of A9
  measures "d108" radius of A10
  measures "d109" radius of A11
extrude "Extrude1'" add sketch "Sketch32" along normal blind 1 separate body contours L0 L1 L2 L3 | L4 A4 L5 A5 L6 A6 L7 A7 L8 L9 L10 L11 A8 A9 A10 A11 makes body 10 in component "Component"
move_body "Move7" bodies 9 to x (1, 0, 0) y (0, 1, 0) z (0, 0, 1) at (0, 0, 2)
sketch "Sketch33" plane through (0, 0, -20) normal (0, 0, 1) x (-1, 0, 0)
  circle A0 centre (-10, -120) radius 1.75
  line L0 (165, -10) -> (5, -10)
  arc A1 (0, -5) -> (5, -10) centre (5, -5) ccw
  line L1 (0, -5) -> (0, 120)
  arc A2 (5, 125) -> (0, 120) centre (5, 120) ccw
  line L2 (5, 125) -> (165, 125)
  arc A3 (170, 120) -> (165, 125) centre (165, 120) ccw
  line L3 (170, 120) -> (170, -5)
  arc A4 (165, -10) -> (170, -5) centre (165, -5) ccw
  circle A5 centre (180, -120) radius 1.75
  circle A6 centre (-10, 130) radius 1.75
  circle A7 centre (180, 130) radius 1.75
  arc A8 (180, -130) -> (190, -120) centre (180, -120) ccw
  line L4 (190, -120) -> (190, 130)
  arc A9 (190, 130) -> (180, 140) centre (180, 130) ccw
  line L5 (180, 140) -> (-10, 140)
  arc A10 (-10, 140) -> (-20, 130) centre (-10, 130) ccw
  line L6 (-20, 130) -> (-20, -120)
  arc A11 (-20, -120) -> (-10, -130) centre (-10, -120) ccw
  line L7 (-10, -130) -> (180, -130)
  circle A12 centre (160, -110) radius 5
  circle A13 centre (10, -110) radius 5
  dimension "d112" = 10
  dimension "d113" = 10
  measures "d112" diameter of A12
  measures "d113" diameter of A13
extrude "Extrude28" add sketch "Sketch33" along normal blind 200 separate body contours A12 | A13 makes body 11 at (-14.9752, 110.4978, 46.6667) makes body 12 at (-164.9752, 110.4978, 46.6667)